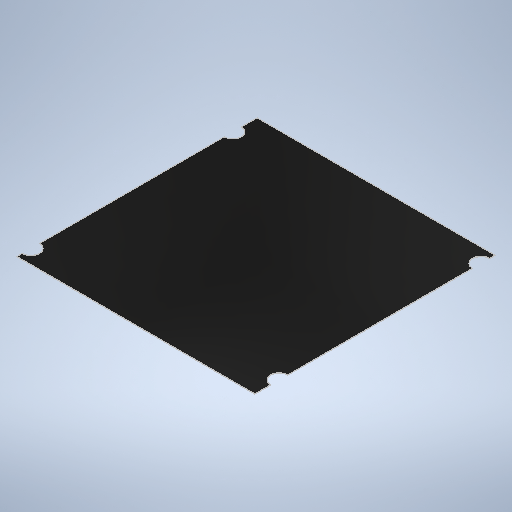
# Autodesk Inventor part: Coverplate Film
Saved by Autodesk Inventor 2025 (Build 290162000, 162)
## iProperties
Created: 2022-02-23
Part Number: Coverplate Film
Material: Thermoplastic Resin
Document SubType Name: Modeling
Designer: Caleb
Density: 1.28 g/cm^3
Appearance: Smooth - Black
Author: Caleb
Autodesk Inventor part; units mm, degrees
ref_plane "YZ Plane" through (0, 0, 0) normal (1, 0, 0) x (0, 1, 0)
ref_plane "XZ Plane" through (0, 0, 0) normal (0, 1, 0) x (-1, 0, 0)
ref_plane "XY Plane" through (0, 0, 0) normal (0, 0, 1) x (1, 0, 0)
sketch "Sketch1" plane through (0, 0, 0) normal (0, 1, 0) x (-1, 0, 0)
  line L0 (-20.8, -21) -> (20.8, -21)
  line L1 (20.8, -21) -> (20.8, 21)
  line L2 (20.8, 21) -> (-20.8, 21)
  line L3 (-20.8, 21) -> (-20.8, -21)
  line L4 (-20.8, -21) -> (20.8, 21) construction
  line L5 (20.8, -21) -> (-20.8, 21) construction
  point P0 (0, 0)
  dimension "d0" = 42
  dimension "d1" = 41.6
  constraints: 12 end point, 2 midpoint, 2 parallel, 1 horizontal, 1 perpendicular
  measures "d0" distance of L0.end L1.end
  measures "d1" distance of L1.end L2.end
extrude "Extrusion1" add sketch "Sketch1" along normal blind 0.08
sketch "Sketch2" plane through (0, 0.08, 0) normal (0, 1, 0) x (1, 0, 0)
  arc A0 (-20.8, 15.25) -> (-20.8, 18.25) centre (-20.8, 16.75) ccw
  line L0 (-20.8, 21) -> (-20.8, -21) projected
  line L1 (20.8, 21) -> (-20.8, 21) projected
  arc A1 (-20.8, -20.05) -> (-20.8, -17.05) centre (-20.8, -18.55) ccw
  line L2 (20.8, -21) -> (20.8, 21) projected
  arc A2 (20.8, 20.05) -> (20.8, 17.05) centre (20.8, 18.55) ccw
  arc A3 (20.8, -15.25) -> (20.8, -18.25) centre (20.8, -16.75) ccw
  line L3 (-20.8, -21) -> (20.8, -21) projected
  line L4 (20.8, -15.25) -> (20.8, -18.25)
  line L5 (20.8, 20.05) -> (20.8, 17.05)
  line L6 (-20.8, 18.25) -> (-20.8, 15.25)
  line L7 (-20.8, -17.05) -> (-20.8, -20.05)
  point P0 (20.8, 12.55)
  point P1 (20.8, -6.06)
  point P2 (20.8, -9.06)
  dimension "d5" = 1.5
  dimension "d8" = 3
  dimension "d9" = 4.25
  dimension "d10" = 1.5
  dimension "d11" = 1.5
  dimension "d12" = 1.5
  dimension "d13" = 39.55
  dimension "d14" = 4.25
  dimension "d15" = 39.55
  constraints: 11 point on line, 9 point on circle, 8 end point, 4 centre point, 3 collinear
  measures "d5" radius of A0
  measures "d8" distance of A0.start L6.start
  measures "d9" distance from line of L1 A0.centre
  measures "d10" radius of A1
  measures "d11" radius of A3
  measures "d12" radius of A2
  measures "d13" distance from line of L1 A1.centre
  measures "d14" distance from line of L3 A3.centre
  measures "d15" distance from line of L3 A2.centre
extrude "Extrusion2" cut sketch "Sketch2" against normal blind 0.08 contours L0 A0 | A1 L0 | L2 A2 | A3 L2
equation "\"d10\" = d5"
equation "\"d11\" = d5"
equation "\"d12\" = d5"
equation "\"d14\" = d9"
equation "\"d15\" = d13"
body "Solid1"
